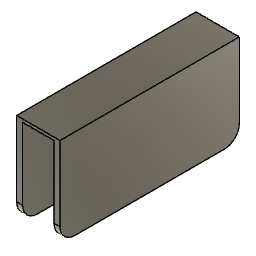
antennabase v1 (Autodesk Fusion 360 design; units mm, degrees)
Autodesk Fusion 360 part; units mm, degrees
sketch "Sketch1" plane through (0, 0, 0) normal (0, 1, 0) x (1, 0, 0)
  line L0 (-18.5178, -25) -> (-4.0178, -25)
  line L1 (-4.0178, -25) -> (-4.0178, 5)
  line L2 (-4.0178, 5) -> (-18.5178, 5)
  line L3 (-18.5178, 5) -> (-18.5178, -25)
  line L4 (-16.5178, 5) -> (-6.0178, 5)
  line L5 (-6.0178, 5) -> (-6.0178, -24)
  line L6 (-6.0178, -24) -> (-16.5178, -24)
  line L7 (-16.5178, -24) -> (-16.5178, 5)
  dimension "d1" = 14.5
  dimension "d2" = 30
  dimension "d3" = 10.5
  dimension "d4" = 2
  dimension "d5" = 1
  constraint horizontal L0
  constraint vertical L1
  constraint horizontal L2
  constraint vertical L3
  constraint horizontal L4
  constraint vertical L5
  constraint horizontal L6
  constraint vertical L7
  constraint coincident L2 L4.start
  measures "d1" distance of L0.start L0.end
  measures "d2" distance of L0.end L1.end
  measures "d3" distance of L4.start L4.end
  measures "d4" distance of L2.end L4.start
  measures "d5" distance of L0 L6.end
extrude "Extrude1" add sketch "Sketch1" along normal blind 60 contours L0 L1 L2 L3 L5 L6 L7
fillet "Fillet1" radius 5 1 edges at (-5.0178, 0, -5)
fillet "Fillet2" radius 5 1 edges at (-17.5178, 0, -5)
fillet "Fillet3" radius 5 1 edges at (-17.5178, 60, -5)
fillet "Fillet4" radius 5 1 edges at (-5.0178, 60, -5)
